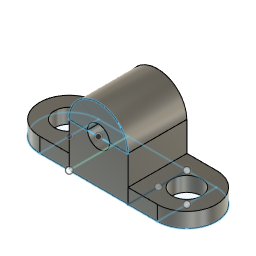
Model 4 v1 (Autodesk Fusion 360 design; units mm, degrees)
Autodesk Fusion 360 part; units mm, degrees
sketch "Sketch1" plane through (0, 0, 0) normal (0, 0, 1) x (1, 0, 0)
  line L0 (19.7933, 40.1491) -> (59.7933, 40.1491)
  line L1 (59.7933, 40.1491) -> (59.7933, 0.1992)
  line L2 (59.7933, 0.1992) -> (19.7933, 0.1992)
  line L3 (19.7933, 0.1992) -> (19.7933, 40.1491)
  line L4 (-0.2067, 40.1993) -> (19.7933, 40.1993)
  line L5 (19.7933, 40.1993) -> (19.7933, 0.1993)
  line L6 (19.7933, 0.1993) -> (-0.2067, 0.1993)
  line L7 (-0.2067, 0.1993) -> (-0.2067, 40.1993)
  line L8 (59.7831, 40.0803) -> (79.7831, 40.0803)
  line L9 (79.7831, 40.0803) -> (79.7831, 0.0803)
  line L10 (79.7831, 0.0803) -> (59.7831, 0.0803)
  line L11 (59.7831, 0.0803) -> (59.7831, 40.0803)
  arc A0 (-0.2067, 40.1993) -> (-0.2067, 0.1993) centre (-0.2067, 20.1993) ccw
  arc A1 (59.7933, 20.7212) -> (59.7933, 19.4394) centre (79.7831, 20.0803) ccw
  arc A2 (79.7831, 0.0803) -> (79.7831, 40.0803) centre (79.7831, 20.0803) ccw
  dimension "d1" = 40
  dimension "d3" = 20
  dimension "d4" = 40
  dimension "d13" = 40
  dimension "d14" = 40
  constraint horizontal L0
  constraint vertical L1
  constraint horizontal L2
  constraint vertical L3
  constraint horizontal L4
  constraint vertical L5
  constraint horizontal L6
  constraint vertical L7
  constraint horizontal L8
  constraint vertical L9
  constraint horizontal L10
  constraint vertical L11
  constraint midpoint L7 A0.centre
  constraint midpoint L9 A1.centre
  constraint coincident L1 A1.start
  constraint coincident L1 A1.end
  constraint concentric A1 A2
  measures "d1" distance of L0.start L0.end
  measures "d3" distance of L4.start L4.end
  measures "d4" distance of L4.start L6.end
  measures "d13" diameter of A0
  measures "d14" diameter of A1
extrude "Extrude1" add sketch "Sketch1" along normal blind 10 contours L3 L4 L5 L6 L7 makes body 1
extrude "Extrude2" add sketch "Sketch1" along normal blind 30 separate body contours L0 L1 L2 L3 L5 L8 L11 makes body 2
extrude "Extrude3" add sketch "Sketch1" along normal blind 10 separate body contours L1 L2 L8 L9 L10 L11 makes body 3
extrude "Extrude4" add sketch "Sketch1" along normal blind 10 contours L7 A0 bodies 1
extrude "Extrude5" add sketch "Sketch1" along normal blind 10 contours L9 A2 bodies 3
hole "Hole1" at (-0.2067, 20.1993, 10) direction (0, 0, -1) diameter 20 depth 20 tip angle 180 bodies 1
hole "Hole2" at (79.7831, 20.0803, 10) direction (0, 0, -1) diameter 20 depth 20 tip angle 180 bodies 3
sketch "Sketch3" plane through (0, 0, 0) normal (0, 1, 0) x (1, 0, 0)
  arc A0 (19.8, -30) -> (59.8, -30) centre (39.8, -29.8598) ccw
  line L0 (19.8, -30) -> (39.8, -29.8598)
  line L1 (39.8, -29.8598) -> (59.8, -30)
  constraint coincident A0.centre L0.end
extrude "Extrude6" add sketch "Sketch3" along normal blind 40 separate body makes body 4
hole "Hole3" at (39.8, 0, 29.8598) direction (0, 1, 0) diameter 15 depth 50 tip angle 180 bodies 2 4
